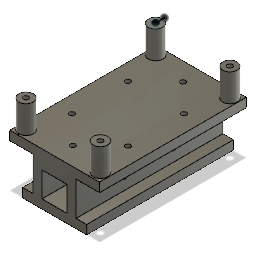
FLIGH_CONTROLLER_BASE v1 (Autodesk Fusion 360 design; units mm, degrees)
Autodesk Fusion 360 part; units mm, degrees
note: some values were not read from the file. Chosen so that the rebuilt part matches the saved one: which bodies a step acts on. Set by a fixed rule: which sketch regions a step uses.
sketch "Sketch1" plane through (0, 0, 0) normal (0, 0, 1) x (1, 0, 0)
  line L0 (0, 0) -> (13.5, 0)
  line L1 (13.5, 0) -> (13.5, 13.5)
  line L2 (13.5, 13.5) -> (0, 13.5)
  line L3 (0, 13.5) -> (0, 0)
  line L4 (-5, -5) -> (18.5, -5)
  line L5 (18.5, -5) -> (18.5, 18.5)
  line L6 (18.5, 18.5) -> (-5, 18.5)
  line L7 (-5, 18.5) -> (-5, -5)
  dimension "d1" = 13.5
  dimension "d2" = 13.5
  dimension "d3" = 5
  constraint horizontal L0
  constraint vertical L1
  constraint horizontal L2
  constraint vertical L3
  constraint coincident L0.start L3.end
  measures "d1" distance of L0.start L2.end
  measures "d2" distance of L0.start L0.end
  measures "d48" distance of L0.start
extrude "Extrude1" add sketch "Sketch1" along normal blind 80 makes body 1
sketch "Sketch2" plane through (0, 0, 80) normal (0, 0, 1) x (1, 0, 0)
  line L0 (0, 0) -> (0, 13.5)
  line L1 (0, 13.5) -> (13.5, 13.5)
  line L2 (13.5, 13.5) -> (13.5, 0)
  line L3 (13.5, 0) -> (0, 0)
  line L4 (-5, 18.5) -> (-5, -5)
  line L5 (-5, -5) -> (18.5, -5)
  line L6 (18.5, -5) -> (18.5, 18.5)
  line L7 (18.5, 18.5) -> (-5, 18.5)
  line L8 (13.5, 0) -> (18.5, 0)
  line L9 (6.75, 0) -> (24.25, 0)
  line L10 (6.75, 0) -> (-10.75, 0)
  line L11 (24.25, 0) -> (24.25, -5)
  line L12 (24.25, -5) -> (18.5, -5)
  line L13 (-10.75, 0) -> (-10.75, -5)
  line L14 (-10.75, -5) -> (-5, -5)
  dimension "d6" = 17.5
  dimension "d7" = 17.5
  constraint coincident L2.end L3.start
  constraint coincident L6 L8.end
  constraint perpendicular L6 L8
  constraint midpoint L3 L9.start
  constraint perpendicular L6 L9
  constraint perpendicular L4 L10
  constraint perpendicular L9 L11
  constraint coincident L5.end L6.start
  constraint perpendicular L10 L13
  constraint coincident L4.end L5.start
  constraint perpendicular L4 L14
  measures "d6" distance of L9.start L9.end
  measures "d7" distance of L9.start L10.end
extrude "Extrude2" add sketch "Sketch2" against normal blind 80 contours L4 L10 L13 L14 | L6 L9 L11 L12 bodies 1
sketch "Sketch3" plane through (0, 18.5, 0) normal (0, 1, 0) x (-1, 0, 0)
  line L0 (-18.5, 0) -> (5, 0)
  line L1 (5, 0) -> (5, 80)
  line L2 (5, 80) -> (-18.5, 80)
  line L3 (-18.5, 80) -> (-18.5, 0)
  line L4 (-6.75, 80) -> (-31.25, 80)
  line L5 (-6.75, 80) -> (17.75, 80)
  line L6 (-6.75, 0) -> (-31.25, 0)
  line L7 (-6.75, 0) -> (17.75, 0)
  line L8 (17.75, 0) -> (17.75, 80)
  line L9 (-31.25, 0) -> (-31.25, 80)
  dimension "d10" = 24.5
  dimension "d11" = 24.5
  dimension "d12" = 24.5
  dimension "d13" = 24.5
  constraint midpoint L2 L4.start
  constraint perpendicular L3 L4
  constraint perpendicular L1 L5
  constraint midpoint L0 L6.start
  constraint parallel L0 L6
  constraint parallel L0 L7
  measures "d10" distance of L4.start L4.end
  measures "d11" distance of L4.start L5.end
  measures "d12" distance of L6.start L6.end
  measures "d13" distance of L6.start L7.end
extrude "Extrude3" add sketch "Sketch3" along normal blind 5 bodies 1
sketch "Sketch4" plane through (0, 23.5, 0) normal (0, 1, 0) x (-1, 0, 0)
  line L0 (-31.25, 0) -> (17.75, 0)
  line L1 (17.75, 0) -> (17.75, 80)
  line L2 (17.75, 80) -> (-31.25, 80)
  line L3 (-31.25, 80) -> (-31.25, 0)
  line L4 (8.5, 24.75) -> (8.5, 55.25)
  line L5 (8.5, 55.25) -> (-22, 55.25)
  line L6 (-22, 55.25) -> (-22, 24.75)
  line L7 (-22, 24.75) -> (8.5, 24.75)
  circle A0 centre (8.5, 55.25) radius 1.35
  circle A1 centre (8.5, 24.75) radius 1.35
  circle A2 centre (-22, 24.75) radius 1.35
  circle A3 centre (-22, 55.25) radius 1.35
  dimension "d18" = 30.5
  dimension "d19" = 30.5
  dimension "d20" = 30.5
  dimension "d21" = 2.7
  dimension "d22" = 2.7
  dimension "d23" = 2.7
  dimension "d24" = 2.7
  constraint perpendicular L4 L5
  constraint perpendicular L5 L6
  constraint coincident L4.end L5.start
  constraint coincident L4.start L7.end
  constraint coincident L6.end L7.start
  constraint coincident L5.end L6.start
  measures "d18" distance of L4.start L4.end
  measures "d19" distance of L4.end L5.end
  measures "d20" distance of L5.end L6.end
  measures "d21" diameter of A0
  measures "d22" diameter of A1
  measures "d23" diameter of A2
  measures "d24" diameter of A3
extrude "Extrude4" cut sketch "Sketch4" against normal blind 15 contours L4 L7 A1 | L4 L7 A1 | L4 L5 A0 | L4 L5 A0 | L6 L7 A2 | L6 L7 A2 | L5 L6 A3 | L5 L6 A3 bodies 1
sketch "Sketch5" plane through (0, 23.5, 0) normal (0, 1, 0) x (-1, 0, 0)
  circle A0 centre (-22, 55.25) radius 1.35
  circle A1 centre (8.5, 55.25) radius 1.35
  circle A2 centre (-22, 24.75) radius 1.35
  circle A3 centre (8.5, 24.75) radius 1.35
  line L0 (-31.25, 0) -> (17.75, 0)
  line L1 (17.75, 0) -> (17.75, 80)
  line L2 (17.75, 80) -> (-31.25, 80)
  line L3 (-31.25, 80) -> (-31.25, 0)
  circle A4 centre (8.5, 55.25) radius 1.5
  circle A5 centre (8.5, 24.75) radius 1.5
  circle A6 centre (-22, 24.75) radius 1.5
  circle A7 centre (-22, 55.25) radius 1.5
  dimension "d27" = 3
  dimension "d28" = 3
  dimension "d29" = 3
  dimension "d30" = 3
  constraint concentric A1 A4
  constraint concentric A3 A5
  constraint concentric A2 A6
  constraint concentric A0 A7
  measures "d27" diameter of A4
  measures "d28" diameter of A5
  measures "d29" diameter of A6
  measures "d30" diameter of A7
extrude "Extrude5" cut sketch "Sketch5" against normal blind 15 contours A4 | A5 | A6 | A7 bodies 1
sketch "Sketch6" plane through (0, 23.5, 0) normal (0, 1, 0) x (-1, 0, 0)
  circle A0 centre (8.5, 55.25) radius 1.5
  circle A1 centre (8.5, 24.75) radius 1.5
  circle A2 centre (-22, 55.25) radius 1.5
  circle A3 centre (-22, 24.75) radius 1.5
  line L0 (-31.25, 0) -> (17.75, 0)
  line L1 (17.75, 0) -> (17.75, 80)
  line L2 (17.75, 80) -> (-31.25, 80)
  line L3 (-31.25, 80) -> (-31.25, 0)
  line L4 (-31.25, 80) -> (-31.25, 75.25)
  line L5 (-27, 75.25) -> (-27, 4.75)
  line L6 (-27, 4.75) -> (13.5, 4.75)
  line L7 (13.5, 4.75) -> (13.5, 75.25)
  line L8 (13.5, 75.25) -> (-27, 75.25)
  circle A4 centre (-27, 75.25) radius 1.5
  circle A5 centre (13.5, 75.25) radius 1.5
  circle A6 centre (13.5, 4.75) radius 1.5
  circle A7 centre (-27, 4.75) radius 1.5
  circle A8 centre (13.5, 4.75) radius 4
  circle A9 centre (13.5, 75.25) radius 4
  circle A10 centre (-27, 75.25) radius 4
  circle A11 centre (-27, 4.75) radius 4
  dimension "d33" = 4.75
  dimension "d34" = 4.25
  dimension "d35" = 70.5
  dimension "d36" = 40.5
  dimension "d37" = 70.5
  dimension "d38" = 3
  dimension "d39" = 3
  dimension "d40" = 3
  dimension "d41" = 3
  dimension "d42" = 8
  dimension "d43" = 8
  dimension "d44" = 8
  dimension "d45" = 8
  constraint coincident L2.end L3.start
  constraint perpendicular L2 L4
  constraint perpendicular L5 L6
  constraint perpendicular L6 L7
  constraint coincident L5.start L8.end
  constraint coincident L7.end L8.start
  constraint coincident L6.end L7.start
  constraint coincident L5.end L6.start
  measures "d33" distance of L2.end L4.end
  measures "d34" distance of L4.end L5.start
  measures "d35" distance of L5.start L5.end
  measures "d36" distance of L5.end L6.end
  measures "d37" distance of L6.end L7.end
  measures "d38" diameter of A4
  measures "d39" diameter of A5
  measures "d40" diameter of A6
  measures "d41" diameter of A7
  measures "d42" diameter of A8
  measures "d43" diameter of A9
  measures "d44" diameter of A10
  measures "d45" diameter of A11
extrude "Extrude6" add sketch "Sketch6" along normal blind 15 contours L5 L8 A4 A10 | L5 L8 A4 A10 | L5 L6 A7 A11 | L5 L6 A7 A11 | L7 L8 A5 A9 | L7 L8 A5 A9 | L6 L7 A6 A8 | L6 L7 A6 A8 bodies 1
sketch "Sketch7" plane through (0, 23.5, 0) normal (0, 1, 0) x (-1, 0, 0)
  circle A0 centre (-27, 4.75) radius 4
  circle A1 centre (13.5, 4.75) radius 4
  circle A2 centre (8.5, 55.25) radius 1.5
  circle A3 centre (8.5, 24.75) radius 1.5
  circle A4 centre (-22, 55.25) radius 1.5
  circle A5 centre (-22, 24.75) radius 1.5
  line L0 (-31.25, 0) -> (17.75, 0)
  line L1 (17.75, 0) -> (17.75, 80)
  line L2 (17.75, 80) -> (-31.25, 80)
  line L3 (-31.25, 80) -> (-31.25, 0)
  circle A6 centre (13.5, 75.25) radius 4
  circle A7 centre (-27, 75.25) radius 4
  line L4 (-6.75, 80) -> (-6.75, 0)
  line L5 (-6.75, 80) -> (-6.75, 70)
  circle A8 centre (-6.75, 70) radius 1.5
  line L6 (-6.75, 70) -> (-6.75, 10)
  circle A9 centre (-6.75, 10) radius 1.5
  circle A10 centre (-6.75, 10) radius 3.5
  circle A11 centre (-6.75, 70) radius 3.5
  dimension "d48" = 10
  dimension "d49" = 3
  dimension "d51" = 3
  dimension "d52" = 10
  dimension "d53" = 7
  dimension "d54" = 7
  constraint midpoint L2 L4.start
  constraint midpoint L0 L4.end
  constraint perpendicular L2 L5
  constraint coincident L5.end A8.centre
  constraint parallel L4 L6
  constraint coincident L6.end A9.centre
  constraint concentric A9 A10
  constraint concentric A8 A11
  measures "d48" distance of L4.start L5.end
  measures "d49" diameter of A8
  measures "d51" diameter of A9
  measures "d52" distance of L0 L6.end
  measures "d53" diameter of A10
  measures "d54" diameter of A11
extrude "Extrude7" add sketch "Sketch7" along normal blind 4 contours L4 L6 A9 A10 | L4 L6 A9 A10 | L4 L5 A8 L6 A11 | L4 L5 A8 L6 A11 bodies 1
extrude "Extrude8" add 2 faces at (9.3664, 27.5, 68.933) (3.9353, 27.5, 10.2484) along direction (0, 1, 0) blind 2 on bodies 1 bodies 1
sketch "Sketch8" plane through (0, 29.5, 0) normal (0, 1, 0) x (-1, 0, 0)
  circle A0 centre (-6.75, 10) radius 1.5
  circle A1 centre (-6.75, 10) radius 3.5
  circle A2 centre (-6.75, 10) radius 2.5
  dimension "d59" = 5
  constraint concentric A0 A2
  measures "d59" diameter of A2
extrude "Extrude9" cut sketch "Sketch8" against normal blind 2 contours A2 bodies 1
sketch "Sketch9" plane through (0, 29.5, 0) normal (0, 1, 0) x (-1, 0, 0)
  circle A0 centre (-6.75, 70) radius 1.5
  circle A1 centre (-6.75, 70) radius 3.5
  circle A2 centre (-6.75, 70) radius 2.75
  dimension "d62" = 5.5
  constraint concentric A0 A2
  measures "d62" diameter of A2
extrude "Extrude10" cut sketch "Sketch9" against normal blind 2 contours A2 bodies 1
sketch "Sketch10" plane through (0, 29.5, 0) normal (0, 1, 0) x (-1, 0, 0)
  circle A0 centre (-6.75, 10) radius 2.5
  circle A1 centre (-6.75, 10) radius 3.5
  circle A2 centre (-6.75, 10) radius 2.75
  dimension "d65" = 5.5
  constraint concentric A0 A2
  measures "d65" diameter of A2
extrude "Extrude11" cut sketch "Sketch10" against normal blind 2 contours A2 bodies 1
extrude "Extrude12" cut 2 faces at (6.8613, 23.5, 68.9492) (7.078, 23.5, 10.4986) along direction (0, -1, 0) blind 8 on bodies 1 bodies 1
sketch "Sketch11" plane through (18.5, 0, 0) normal (1, 0, 0) x (0, 0, -1)
  line L0 (-80, 0) -> (0, 0)
  line L1 (0, 0) -> (0, 18.5)
  line L2 (0, 18.5) -> (-80, 18.5)
  line L3 (-80, 18.5) -> (-80, 0)
  line L4 (-80, 0) -> (-80, 6.75)
  line L5 (-80, 6.75) -> (0, 6.75)
  line L6 (-80, 6.75) -> (-53.3333, 6.75)
  line L7 (0, 6.75) -> (-26.6667, 6.75)
  circle A0 centre (-53.3333, 6.75) radius 1.5
  circle A1 centre (-26.6667, 6.75) radius 1.5
  dimension "d70" = 6.75
  dimension "d71" = 26.6667
  dimension "d72" = 26.6667
  dimension "d73" = 3
  dimension "d74" = 3
  constraint coincident L0.start L3.end
  constraint perpendicular L0 L4
  constraint coincident L1 L5.end
  constraint perpendicular L1 L5
  constraint perpendicular L3 L6
  constraint perpendicular L1 L7
  constraint coincident L6.end A0.centre
  constraint coincident L7.end A1.centre
  measures "d70" distance of L0.start L4.end
  measures "d71" distance of L4.end L6.end
  measures "d72" distance of L5.end L7.end
  measures "d73" diameter of A0
  measures "d74" diameter of A1
extrude "Extrude13" cut sketch "Sketch11" against normal blind 65 contours L5 L6 A0 | L5 L6 A0 | L5 L7 A1 | L5 L7 A1 bodies 1
sketch "Sketch12" plane through (-5, 0, 0) normal (-1, 0, 0) x (0, 0, 1)
  circle A0 centre (53.3333, 6.75) radius 1.5
  circle A1 centre (26.6667, 6.75) radius 1.5
  line L0 (0, 0) -> (80, 0)
  line L1 (80, 0) -> (80, 18.5)
  line L2 (80, 18.5) -> (0, 18.5)
  line L3 (0, 18.5) -> (0, 0)
  line L4 (26.6667, 18.5) -> (26.6667, 13.5)
  line L5 (26.6667, 13.5) -> (26.6667, 15)
  line L6 (26.6667, 15) -> (37.6667, 15)
  line L7 (26.6667, 15) -> (15.6667, 15)
  line L8 (15.6667, 15) -> (15.6667, 18)
  line L9 (15.6667, 18) -> (26.6667, 18)
  line L10 (40, 0) -> (40, 18.5)
  line L11 (53.3333, 15) -> (64.3333, 15)
  line L12 (64.3333, 15) -> (64.3333, 18)
  line L13 (64.3333, 18) -> (53.3333, 18)
  line L14 (53.3333, 18.5) -> (53.3333, 13.5)
  dimension "d77" = 11
  dimension "d78" = 11
  dimension "d79" = 3
  constraint coincident L2 L4.start
  constraint perpendicular L2 L4
  constraint coincident L4 L5.end
  constraint perpendicular L4 L6
  constraint perpendicular L5 L7
  constraint perpendicular L7 L8
  constraint coincident L4 L9.end
  constraint perpendicular L4 L9
  constraint midpoint L0 L10.start
  constraint midpoint L2 L10.end
  constraint symmetric L4.start L10 L14.start
  constraint symmetric L4.end L10 L14.end
  constraint symmetric L5.end L10 L11.start
  constraint symmetric L7.end L10 L11.end
  constraint symmetric L8.end L10 L12.end
  constraint symmetric L9.end L10 L13.end
  measures "d77" distance of L5.end L6.end
  measures "d78" distance of L5.end L7.end
  measures "d79" distance of L7.end L8.end
extrude "Extrude14" cut sketch "Sketch12" against normal blind 45 contours L4 L7 L8 L9 | L11 L12 L13 L14 bodies 1
sketch "Sketch13" plane through (0, 0, 80) normal (0, 0, 1) x (1, 0, 0)
  line L0 (0, 0) -> (0, 13.5)
  line L1 (0, 13.5) -> (13.5, 13.5)
  line L2 (13.5, 13.5) -> (13.5, 0)
  line L3 (13.5, 0) -> (0, 0)
  line L4 (-5, 18.5) -> (-5, 0)
  line L5 (-5, 0) -> (-10.75, 0)
  line L6 (-10.75, 0) -> (-10.75, -5)
  line L7 (-10.75, -5) -> (18.5, -5)
  line L8 (18.5, -5) -> (24.25, -5)
  line L9 (24.25, -5) -> (24.25, 0)
  line L10 (24.25, 0) -> (18.5, 0)
  line L11 (18.5, 0) -> (18.5, 18.5)
  line L12 (18.5, 18.5) -> (31.25, 18.5)
  line L13 (31.25, 18.5) -> (31.25, 23.5)
  line L14 (31.25, 23.5) -> (-17.75, 23.5)
  line L15 (-17.75, 23.5) -> (-17.75, 18.5)
  line L16 (-17.75, 18.5) -> (-5, 18.5)
  line L17 (13.575, -0.075) -> (-0.075, -0.075)
  line L18 (-0.075, -0.075) -> (-0.075, 13.575)
  line L19 (-0.075, 13.575) -> (13.575, 13.575)
  line L20 (13.575, 13.575) -> (13.575, -0.075)
  dimension "d82" = -0.075
extrude "Extrude15" cut sketch "Sketch13" against normal blind 100 contours L17 L18 L19 L20 bodies 1
sketch "Sketch14" plane through (-5, 0, 0) normal (-1, 0, 0) x (0, 0, 1)
  line L0 (26.6667, 15) -> (15.6667, 15)
  line L1 (15.6667, 15) -> (15.6667, 18)
  line L2 (15.6667, 18) -> (26.6667, 18)
  line L3 (26.6667, 18) -> (26.6667, 15)
  line L4 (53.3333, 15) -> (53.3333, 18)
  line L5 (53.3333, 18) -> (64.3333, 18)
  line L6 (64.3333, 18) -> (64.3333, 15)
  line L7 (64.3333, 15) -> (53.3333, 15)
  circle A0 centre (53.3333, 6.75) radius 1.5
  circle A1 centre (26.6667, 6.75) radius 1.5
  line L8 (0, 0) -> (80, 0)
  line L9 (80, 0) -> (80, 18.5)
  line L10 (80, 18.5) -> (0, 18.5)
  line L11 (0, 18.5) -> (0, 0)
  circle A2 centre (26.6667, 6.75) radius 1.45
  circle A3 centre (53.3333, 6.75) radius 1.45
  dimension "d85" = 2.9
  dimension "d86" = 2.9
  constraint concentric A1 A2
  constraint concentric A0 A3
  measures "d85" diameter of A2
  measures "d86" diameter of A3
extrude "Extrude16" add sketch "Sketch14" against normal blind 23.5 contours A0 | A1 bodies 1
sketch "Sketch15" plane through (0, 0, 0) normal (0, 0, -1) x (-1, 0, 0)
  line L0 (0.075, 13.575) -> (0.075, -0.075)
  line L1 (0.075, -0.075) -> (-13.575, -0.075)
  line L2 (-13.575, -0.075) -> (-13.575, 13.575)
  line L3 (-13.575, 13.575) -> (0.075, 13.575)
  line L4 (5, 0) -> (5, 18.5)
  line L5 (5, 18.5) -> (17.75, 18.5)
  line L6 (17.75, 18.5) -> (17.75, 23.5)
  line L7 (17.75, 23.5) -> (-31.25, 23.5)
  line L8 (-31.25, 23.5) -> (-31.25, 18.5)
  line L9 (-31.25, 18.5) -> (-18.5, 18.5)
  line L10 (-18.5, 18.5) -> (-18.5, 0)
  line L11 (-18.5, 0) -> (-24.25, 0)
  line L12 (-24.25, 0) -> (-24.25, -5)
  line L13 (-24.25, -5) -> (-18.5, -5)
  line L14 (-18.5, -5) -> (10.75, -5)
  line L15 (10.75, -5) -> (10.75, 0)
  line L16 (10.75, 0) -> (5, 0)
  line L17 (-13.575, 13.575) -> (0.075, 13.575)
  line L18 (0.075, 13.575) -> (0.075, -0.075)
  line L19 (0.075, -0.075) -> (-13.575, -0.075)
  line L20 (-13.575, -0.075) -> (-13.575, 13.575)
  constraint horizontal L17
  constraint vertical L18
  constraint horizontal L19
  constraint vertical L20
  constraint coincident L0.end L1.start
  constraint coincident L2.end L3.start
extrude "Extrude17" cut sketch "Sketch15" against normal blind 91 contours L0 L1 L2 L3 L17 L18 L19 L20 bodies 1
sketch "Sketch16" plane through (0, 23.5, 0) normal (0, 1, 0) x (-1, 0, 0)
  circle A0 centre (-6.75, 70) radius 3.5
  circle A1 centre (-27, 4.75) radius 4
  circle A2 centre (13.5, 4.75) radius 4
  circle A3 centre (8.5, 55.25) radius 1.5
  circle A4 centre (8.5, 24.75) radius 1.5
  circle A5 centre (-22, 55.25) radius 1.5
  circle A6 centre (-22, 24.75) radius 1.5
  line L0 (-31.25, 0) -> (17.75, 0)
  line L1 (17.75, 0) -> (17.75, 80)
  line L2 (17.75, 80) -> (-31.25, 80)
  line L3 (-31.25, 80) -> (-31.25, 0)
  circle A7 centre (13.5, 75.25) radius 4
  circle A8 centre (-27, 75.25) radius 4
  circle A9 centre (-6.75, 10) radius 3.5
  circle A10 centre (8.5, 24.75) radius 1.2
  circle A11 centre (8.5, 55.25) radius 1.2
  circle A12 centre (-22, 55.25) radius 1.2
  circle A13 centre (-22, 24.75) radius 1.2
  circle A14 centre (13.5, 4.75) radius 1.2
  circle A15 centre (-27, 4.75) radius 1.2
  circle A16 centre (-27, 75.25) radius 1.2
  circle A17 centre (13.5, 75.25) radius 1.2
  circle A18 centre (13.5, 75.25) radius 1.5
  circle A19 centre (-27, 75.25) radius 1.5
  circle A20 centre (-27, 4.75) radius 1.5
  circle A21 centre (13.5, 4.75) radius 1.5
  dimension "d91" = 2.4
  dimension "d92" = 2.4
  dimension "d93" = 2.4
  dimension "d94" = 2.4
  dimension "d95" = 2.4
  dimension "d96" = 2.4
  dimension "d97" = 2.4
  dimension "d98" = 2.4
  dimension "d99" = 3
  dimension "d100" = 3
  dimension "d101" = 3
  dimension "d102" = 3
  constraint concentric A4 A10
  constraint concentric A3 A11
  constraint concentric A5 A12
  constraint concentric A6 A13
  constraint concentric A2 A14
  constraint concentric A1 A15
  constraint concentric A8 A16
  constraint concentric A7 A17
  constraint concentric A17 A18
  constraint concentric A16 A19
  constraint concentric A15 A20
  constraint concentric A14 A21
  measures "d91" diameter of A10
  measures "d92" diameter of A11
  measures "d93" diameter of A12
  measures "d94" diameter of A13
  measures "d95" diameter of A14
  measures "d96" diameter of A15
  measures "d97" diameter of A16
  measures "d98" diameter of A17
  measures "d99" diameter of A18
  measures "d100" diameter of A19
  measures "d101" diameter of A20
  measures "d102" diameter of A21
extrude "Extrude18" cut sketch "Sketch16" against normal blind 10 contours A18 | A19 | A20 | A21 bodies 1 makes body 2 at (25.806, 21.8333, 4.6305) makes body 3 at (-14.694, 21.8333, 4.6305) makes body 4 at (25.8015, 21.8333, 75.3098) makes body 5 at (2.0332, 23.5, 35.2568)
extrude "Extrude19" cut 4 faces at (27.4274, 18.5, 74.9373) (-12.7396, 18.5, 75.0764) (-13.7494, 18.5, 5.2985) (27.089, 18.5, 5.14) along direction (0, 1, 0) blind 40 on bodies 1 2 3 4 bodies 1 2 3 4
sketch "Sketch17" plane through (0, 23.5, 0) normal (0, 1, 0) x (-1, 0, 0)
  circle A0 centre (-6.75, 70) radius 3.5
  circle A1 centre (-27, 4.75) radius 4
  circle A2 centre (13.5, 4.75) radius 4
  circle A3 centre (8.5, 55.25) radius 1.5
  circle A4 centre (8.5, 24.75) radius 1.5
  circle A5 centre (-22, 55.25) radius 1.5
  circle A6 centre (-22, 24.75) radius 1.5
  line L0 (-31.25, 0) -> (17.75, 0)
  line L1 (17.75, 0) -> (17.75, 80)
  line L2 (17.75, 80) -> (-31.25, 80)
  line L3 (-31.25, 80) -> (-31.25, 0)
  circle A7 centre (13.5, 75.25) radius 4
  circle A8 centre (-27, 75.25) radius 4
  circle A9 centre (-6.75, 10) radius 3.5
  circle A10 centre (8.5, 55.25) radius 1.2
  circle A11 centre (-22, 55.25) radius 1.2
  circle A12 centre (-22, 24.75) radius 1.2
  circle A13 centre (8.5, 24.75) radius 1.2
  dimension "d107" = 2.4
  dimension "d108" = 2.4
  dimension "d109" = 2.4
  dimension "d110" = 2.4
  constraint concentric A3 A10
  constraint concentric A5 A11
  constraint concentric A6 A12
  constraint concentric A4 A13
  measures "d107" diameter of A10
  measures "d108" diameter of A11
  measures "d109" diameter of A12
  measures "d110" diameter of A13
extrude "Extrude20" add sketch "Sketch17" against normal blind 5 contours A3 | A4 | A5 | A6 bodies 1 2 3 4 5
sketch "Sketch18" plane through (0, 38.5, 0) normal (0, 1, 0) x (-1, 0, 0)
  circle A0 centre (-27, 75.25) radius 1.5
  circle A1 centre (-27, 75.25) radius 4
  circle A2 centre (-27, 75.25) radius 1.2
  dimension "d113" = 2.4
  constraint concentric A0 A2
  measures "d113" diameter of A2
extrude "Extrude21" add sketch "Sketch18" against normal blind 20 contours A0 bodies 1
sketch "Sketch19" plane through (0, 38.5, 0) normal (0, 1, 0) x (-1, 0, 0)
  circle A0 centre (13.5, 75.25) radius 1.5
  circle A1 centre (13.5, 75.25) radius 4
  circle A2 centre (13.5, 75.25) radius 1.2
  dimension "d116" = 2.4
  constraint concentric A0 A2
  measures "d116" diameter of A2
extrude "Extrude22" add sketch "Sketch19" against normal blind 20 contours A0 bodies 1
sketch "Sketch20" plane through (0, 38.5, 0) normal (0, 1, 0) x (-1, 0, 0)
  circle A0 centre (13.5, 4.75) radius 1.5
  circle A1 centre (13.5, 4.75) radius 4
  circle A2 centre (13.5, 4.75) radius 1.2
  dimension "d119" = 2.4
  constraint concentric A0 A2
  measures "d119" diameter of A2
extrude "Extrude23" add sketch "Sketch20" against normal blind 20 contours A0 bodies 1
sketch "Sketch21" plane through (0, 38.5, 0) normal (0, 1, 0) x (-1, 0, 0)
  circle A0 centre (-27, 4.75) radius 1.5
  circle A1 centre (-27, 4.75) radius 4
  circle A2 centre (-27, 4.75) radius 1.2
  dimension "d122" = 2.4
  constraint concentric A0 A2
  measures "d122" diameter of A2
extrude "Extrude24" add sketch "Sketch21" against normal blind 20 contours A0 bodies 1
sketch "Sketch22" plane through (0, 0, 80) normal (0, 0, 1) x (1, 0, 0)
  line L0 (-0.075, -0.075) -> (-0.075, 13.575)
  line L1 (-0.075, 13.575) -> (13.575, 13.575)
  line L2 (13.575, 13.575) -> (13.575, -0.075)
  line L3 (13.575, -0.075) -> (-0.075, -0.075)
  line L4 (-5, 18.5) -> (-5, 0)
  line L5 (-5, 0) -> (-10.75, 0)
  line L6 (-10.75, 0) -> (-10.75, -5)
  line L7 (-10.75, -5) -> (18.5, -5)
  line L8 (18.5, -5) -> (24.25, -5)
  line L9 (24.25, -5) -> (24.25, 0)
  line L10 (24.25, 0) -> (18.5, 0)
  line L11 (18.5, 0) -> (18.5, 18.5)
  line L12 (18.5, 18.5) -> (31.25, 18.5)
  line L13 (31.25, 18.5) -> (31.25, 23.5)
  line L14 (31.25, 23.5) -> (-17.75, 23.5)
  line L15 (-17.75, 23.5) -> (-17.75, 18.5)
  line L16 (-17.75, 18.5) -> (-5, 18.5)
  line L17 (-1.9861, 23.5) -> (16.1126, 23.5)
  line L18 (16.1126, 23.5) -> (16.1126, 33.7803)
  line L19 (16.1126, 33.7803) -> (-1.9861, 33.7803)
  line L20 (-1.9861, 33.7803) -> (-1.9861, 23.5)
  constraint horizontal L17
  constraint vertical L18
  constraint horizontal L19
  constraint vertical L20
  constraint coincident L14 L17.start
extrude "Extrude25" cut sketch "Sketch22" against normal blind 130 contours L14 L17 L18 L19 L20 bodies 1
sketch "Sketch23" plane through (0, 23.5, 0) normal (0, 1, 0) x (-1, 0, 0)
  circle A0 centre (-6.75, 70) radius 1.5
  circle A1 centre (-6.75, 10) radius 1.5
  circle A2 centre (-22, 24.75) radius 1.2
  circle A3 centre (-27, 4.75) radius 4
  circle A4 centre (-27, 75.25) radius 4
  circle A5 centre (-22, 55.25) radius 1.2
  line L0 (-31.25, 0) -> (17.75, 0)
  line L1 (17.75, 0) -> (17.75, 80)
  line L2 (17.75, 80) -> (-31.25, 80)
  line L3 (-31.25, 80) -> (-31.25, 0)
  circle A6 centre (8.5, 24.75) radius 1.2
  circle A7 centre (8.5, 55.25) radius 1.2
  circle A8 centre (13.5, 75.25) radius 4
  circle A9 centre (13.5, 4.75) radius 4
  circle A10 centre (-6.75, 70) radius 1.2
  circle A11 centre (-6.75, 10) radius 1.2
  dimension "d127" = 2.4
  dimension "d128" = 2.4
  constraint concentric A0 A10
  constraint concentric A1 A11
  measures "d127" diameter of A10
  measures "d128" diameter of A11
extrude "Extrude26" add sketch "Sketch23" against normal blind 8 contours A0 | A1 bodies 1
extrude "Extrude27" cut 2 faces at (5.9678, 15.5, 69.8821) (6.726, 15.5, 10.3199) along direction (0, -1, 0) blind 5 on bodies 1 bodies 1
sketch "Sketch24" plane through (18.5, 0, 0) normal (1, 0, 0) x (0, 0, -1)
  circle A0 centre (-26.6667, 6.75) radius 1.45
  circle A1 centre (-53.3333, 6.75) radius 1.45
  line L0 (-15.6667, 15) -> (-26.6667, 15)
  line L1 (-26.6667, 15) -> (-26.6667, 18)
  line L2 (-26.6667, 18) -> (-15.6667, 18)
  line L3 (-15.6667, 18) -> (-15.6667, 15)
  line L4 (-53.3333, 18) -> (-53.3333, 15)
  line L5 (-53.3333, 15) -> (-64.3333, 15)
  line L6 (-64.3333, 15) -> (-64.3333, 18)
  line L7 (-64.3333, 18) -> (-53.3333, 18)
  line L8 (-80, 0) -> (0, 0)
  line L9 (0, 0) -> (0, 18.5)
  line L10 (0, 18.5) -> (-80, 18.5)
  line L11 (-80, 18.5) -> (-80, 0)
  line L12 (-64.3333, 15) -> (-64.3333, 18.5)
  line L13 (-53.3333, 15) -> (-53.3333, 18.5)
  line L14 (-53.3333, 18.5) -> (-64.3333, 18.5)
  constraint coincident L5.end L6.start
  constraint coincident L10 L12.end
  constraint perpendicular L10 L12
  constraint coincident L4.end L5.start
  constraint coincident L10 L13.end
  constraint perpendicular L10 L13
extrude "Extrude28" cut sketch "Sketch24" against normal blind 26 contours L7 L10 L12 L13 L14 bodies 1
sketch "Sketch25" plane through (18.5, 0, 0) normal (1, 0, 0) x (0, 0, -1)
  line L0 (-64.3333, 15) -> (-64.3333, 18.5)
  line L1 (-64.3333, 18.5) -> (-80, 18.5)
  line L2 (-80, 18.5) -> (-80, 0)
  line L3 (-80, 0) -> (0, 0)
  line L4 (0, 0) -> (0, 18.5)
  line L5 (0, 18.5) -> (-53.3333, 18.5)
  line L6 (-53.3333, 18.5) -> (-53.3333, 15)
  line L7 (-53.3333, 15) -> (-64.3333, 15)
  circle A0 centre (-26.6667, 6.75) radius 1.45
  circle A1 centre (-53.3333, 6.75) radius 1.45
  line L8 (-15.6667, 15) -> (-26.6667, 15)
  line L9 (-26.6667, 15) -> (-26.6667, 18)
  line L10 (-26.6667, 18) -> (-15.6667, 18)
  line L11 (-15.6667, 18) -> (-15.6667, 15)
  line L12 (-26.6667, 15) -> (-26.6667, 18.5)
  line L13 (-15.6667, 15) -> (-15.6667, 18.5)
  line L14 (-15.6667, 18.5) -> (-26.6667, 18.5)
  constraint coincident L8.end L9.start
  constraint midpoint L5 L12.end
  constraint coincident L8.start L11.end
  constraint coincident L5 L13.end
  constraint perpendicular L5 L13
extrude "Extrude29" cut sketch "Sketch25" against normal blind 27 contours L5 L10 L12 L13 L14 bodies 1
sketch "Sketch26" plane through (-5, 0, 0) normal (-1, 0, 0) x (0, 0, 1)
  line L0 (26.6667, 18.5) -> (26.6667, 15)
  line L1 (26.6667, 15) -> (15.6667, 15)
  line L2 (15.6667, 15) -> (15.6667, 18)
  line L3 (15.6667, 18) -> (15.6667, 18.5)
  line L4 (15.6667, 18.5) -> (0, 18.5)
  line L5 (0, 18.5) -> (0, 0)
  line L6 (0, 0) -> (80, 0)
  line L7 (80, 0) -> (80, 18.5)
  line L8 (80, 18.5) -> (64.3333, 18.5)
  line L9 (64.3333, 18.5) -> (64.3333, 15)
  line L10 (64.3333, 15) -> (53.3333, 15)
  line L11 (53.3333, 15) -> (53.3333, 18.5)
  line L12 (53.3333, 18.5) -> (26.6667, 18.5)
  circle A0 centre (26.6667, 6.75) radius 1.45
  circle A1 centre (53.3333, 6.75) radius 1.45
sketch "Sketch27" plane through (0, 18.5, 0) normal (0, -1, 0) x (1, 0, 0)
  line L0 (-5, 26.6667) -> (-5, 53.3333)
  line L1 (-5, 53.3333) -> (18.5, 53.3333)
  line L2 (18.5, 53.3333) -> (18.5, 26.6667)
  line L3 (18.5, 26.6667) -> (18.5, 15.6667)
  line L4 (18.5, 15.6667) -> (18.5, 0)
  line L5 (18.5, 0) -> (31.25, 0)
  line L6 (31.25, 0) -> (31.25, 80)
  line L7 (31.25, 80) -> (18.5, 80)
  line L8 (18.5, 80) -> (18.5, 64.3333)
  line L9 (18.5, 64.3333) -> (-5, 64.3333)
  line L10 (-5, 64.3333) -> (-5, 80)
  line L11 (-5, 80) -> (-17.75, 80)
  line L12 (-17.75, 80) -> (-17.75, 0)
  line L13 (-17.75, 0) -> (-5, 0)
  line L14 (-5, 0) -> (-5, 15.6667)
  line L15 (-5, 15.6667) -> (-5, 26.6667)
  circle A0 centre (-8.5, 24.75) radius 1.2
  circle A1 centre (-13.5, 75.25) radius 1.2
  circle A2 centre (-13.5, 4.75) radius 1.2
  circle A3 centre (-8.5, 55.25) radius 1.2
  circle A4 centre (27, 4.75) radius 1.2
  circle A5 centre (27, 75.25) radius 1.2
  circle A6 centre (22, 55.25) radius 1.2
  circle A7 centre (22, 24.75) radius 1.2
  circle A8 centre (27, 4.75) radius 1.4
  circle A9 centre (-13.5, 4.75) radius 1.4
  circle A10 centre (-13.5, 75.25) radius 1.4
  circle A11 centre (27, 75.25) radius 1.4
  dimension "d137" = 2.8
  dimension "d138" = 2.8
  dimension "d139" = 2.8
  dimension "d140" = 2.8
  constraint concentric A4 A8
  constraint concentric A2 A9
  constraint concentric A1 A10
  constraint concentric A5 A11
  measures "d137" diameter of A8
  measures "d138" diameter of A9
  measures "d139" diameter of A10
  measures "d140" diameter of A11
extrude "Extrude30" cut sketch "Sketch27" against normal blind 35 contours A8 | A9 | A10 | A11 bodies 1
sketch "Sketch28" plane through (0, 23.5, 0) normal (0, 1, 0) x (-1, 0, 0)
  circle A0 centre (-6.75, 70) radius 1.2
  circle A1 centre (-6.75, 10) radius 1.2
  circle A2 centre (-22, 24.75) radius 1.2
  circle A3 centre (-27, 4.75) radius 4
  circle A4 centre (-27, 75.25) radius 4
  circle A5 centre (-22, 55.25) radius 1.2
  line L0 (-31.25, 0) -> (17.75, 0)
  line L1 (17.75, 0) -> (17.75, 80)
  line L2 (17.75, 80) -> (-31.25, 80)
  line L3 (-31.25, 80) -> (-31.25, 0)
  circle A6 centre (8.5, 24.75) radius 1.2
  circle A7 centre (8.5, 55.25) radius 1.2
  circle A8 centre (13.5, 75.25) radius 4
  circle A9 centre (13.5, 4.75) radius 4
  circle A10 centre (8.5, 24.75) radius 1.4
  circle A11 centre (8.5, 55.25) radius 1.4
  circle A12 centre (-22, 55.25) radius 1.4
  circle A13 centre (-22, 24.75) radius 1.4
  dimension "d143" = 2.8
  dimension "d144" = 2.8
  dimension "d145" = 2.8
  dimension "d146" = 2.8
  constraint concentric A6 A10
  constraint concentric A7 A11
  constraint concentric A5 A12
  constraint concentric A2 A13
  measures "d143" diameter of A10
  measures "d144" diameter of A11
  measures "d145" diameter of A12
  measures "d146" diameter of A13
extrude "Extrude31" cut sketch "Sketch28" against normal blind 5 contours A10 | A11 | A12 | A13 bodies 1
sketch "Sketch29" plane through (0, 23.5, 0) normal (0, 1, 0) x (-1, 0, 0)
  circle A0 centre (8.5, 24.75) radius 1.4
  circle A1 centre (8.5, 55.25) radius 1.4
  circle A2 centre (-22, 24.75) radius 1.4
  circle A3 centre (-22, 55.25) radius 1.4
  circle A4 centre (-6.75, 70) radius 1.2
  circle A5 centre (-6.75, 10) radius 1.2
  circle A6 centre (-27, 4.75) radius 4
  circle A7 centre (-27, 75.25) radius 4
  line L0 (-31.25, 0) -> (17.75, 0)
  line L1 (17.75, 0) -> (17.75, 80)
  line L2 (17.75, 80) -> (-31.25, 80)
  line L3 (-31.25, 80) -> (-31.25, 0)
  circle A8 centre (13.5, 75.25) radius 4
  circle A9 centre (13.5, 4.75) radius 4
  circle A10 centre (-6.75, 10) radius 1.4
  circle A11 centre (-6.75, 70) radius 1.4
  dimension "d149" = 2.8
  dimension "d150" = 2.8
  constraint concentric A5 A10
  constraint concentric A4 A11
  measures "d149" diameter of A10
  measures "d150" diameter of A11
extrude "Extrude32" cut sketch "Sketch29" against normal blind 15 contours A10 | A11 bodies 1
sketch "Sketch30" plane through (18.5, 0, 0) normal (1, 0, 0) x (0, 0, -1)
  line L0 (-26.6667, 15) -> (-26.6667, 18.5)
  line L1 (-26.6667, 18.5) -> (-53.3333, 18.5)
  line L2 (-53.3333, 18.5) -> (-53.3333, 15)
  line L3 (-53.3333, 15) -> (-64.3333, 15)
  line L4 (-64.3333, 15) -> (-64.3333, 18.5)
  line L5 (-64.3333, 18.5) -> (-80, 18.5)
  line L6 (-80, 18.5) -> (-80, 0)
  line L7 (-80, 0) -> (0, 0)
  line L8 (0, 0) -> (0, 18.5)
  line L9 (0, 18.5) -> (-15.6667, 18.5)
  line L10 (-15.6667, 18.5) -> (-15.6667, 18)
  line L11 (-15.6667, 18) -> (-15.6667, 15)
  line L12 (-15.6667, 15) -> (-26.6667, 15)
  circle A0 centre (-26.6667, 6.75) radius 1.45
  circle A1 centre (-53.3333, 6.75) radius 1.45
  line L13 (-53.3333, 15) -> (-42.3333, 15)
  line L14 (-26.6667, 15) -> (-37.6667, 15)
  line L15 (-42.3333, 15) -> (-42.3333, 18.5)
  line L16 (-37.6667, 15) -> (-37.6667, 18.5)
  dimension "d153" = 11
  dimension "d154" = 11
  constraint coincident L2.end L3.start
  constraint perpendicular L2 L13
  constraint coincident L0.start L12.end
  constraint perpendicular L0 L14
  constraint coincident L1 L15.end
  constraint perpendicular L1 L15
  constraint coincident L1 L16.end
  constraint perpendicular L1 L16
  measures "d153" distance of L2.end L13.end
  measures "d154" distance of L0.start L14.end
extrude "Extrude33" cut sketch "Sketch30" against normal blind 28 contours L0 L1 L14 L16 | L1 L2 L13 L15 bodies 1
sketch "Sketch31" plane through (0, 38.5, 0) normal (0, 1, 0) x (-1, 0, 0)
  circle A0 centre (13.5, 4.75) radius 1.4
  circle A1 centre (13.5, 4.75) radius 4
  line L0 (13.5, 4.75) -> (13.5, 0)
  dimension "d157" = 4.75
  constraint coincident A0.centre A1.centre
  constraint vertical L0
  measures "d157" distance of A0.centre L0.end
equation "d6 = ( 35 / 2 ) * 1 mm"
equation "d7 = ( 35 / 2 ) * 1 mm"
equation "d10 = ( 49 / 2 ) * 1 mm"
equation "d11 = ( 49 / 2 ) * 1 mm"
equation "d12 = ( 49 / 2 ) * 1 mm"
equation "d13 = ( 49 / 2 ) * 1 mm"
equation "d70 = ( 13.5 / 2 ) * 1 mm"
equation "d71 = ( 80 / 3 ) * 1 mm"
equation "d72 = ( 80 / 3 ) * 1 mm"
equation "d82 = ( -0.15 / 2 ) * 1 mm"
